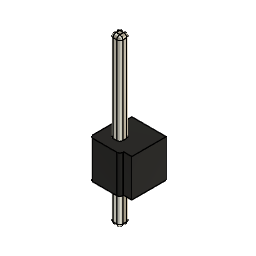
Parametric_Male (Autodesk Fusion 360 design; units mm, degrees)
Autodesk Fusion 360 part; units mm, degrees
sketch "Sketch1" plane through (0, 0, 0) normal (0, 0, 1) x (1, 0, 0)
  line L0 (1, -1) -> (-1, -1)
  line L1 (-1, -1) -> (-1, 1)
  line L2 (-1, 1) -> (1, 1)
  line L3 (1, 1) -> (1, -1)
  line L4 (1, -1) -> (-1, 1) construction
  line L5 (-1, -1) -> (1, 1) construction
  line L6 (0.325, -0.325) -> (-0.325, -0.325)
  line L7 (-0.325, -0.325) -> (-0.325, 0.325)
  line L8 (-0.325, 0.325) -> (0.325, 0.325)
  line L9 (0.325, 0.325) -> (0.325, -0.325)
  line L10 (0.325, -0.325) -> (-0.325, 0.325) construction
  line L11 (-0.325, -0.325) -> (0.325, 0.325) construction
  line L12 (1, 0.75) -> (1.54, 0.75)
  line L13 (1.54, 0.75) -> (1.54, -0.75)
  line L14 (1.54, -0.75) -> (1, -0.75)
  line L15 (1, -0.75) -> (1, 0.75)
  line L16 (-0.75, 1) -> (0.75, 1)
  line L17 (0.75, 1) -> (0.75, 1.54)
  line L18 (0.75, 1.54) -> (-0.75, 1.54)
  line L19 (-0.75, 1.54) -> (-0.75, 1)
  line L20 (0.75, 1.54) -> (1.54, 1.54)
  line L21 (1.54, 1.54) -> (1.54, 0.75)
  dimension "d1" = 2
  dimension "d2" = 2
  dimension "d5" = 0.65
  dimension "d6" = 0.65
  dimension "d13" = 0.54
  dimension "d14" = 0.25
  dimension "d15" = 0.25
  dimension "d16" = 0.54
  dimension "d17" = 0.25
  dimension "d18" = 0.25
  constraint horizontal L0
  constraint perpendicular L0 L1
  constraint parallel L0 L2
  constraint parallel L1 L3
  constraint coincident L4 origin
  constraint coincident L5 origin
  constraint horizontal L6
  constraint perpendicular L6 L7
  constraint parallel L6 L8
  constraint parallel L7 L9
  constraint coincident L10 origin
  constraint coincident L11 origin
  constraint horizontal L12
  constraint vertical L13
  constraint horizontal L14
  constraint vertical L15
  constraint coincident L3 L12.start
  constraint horizontal L16
  constraint vertical L17
  constraint horizontal L18
  constraint vertical L19
  constraint coincident L2 L16.start
  constraint perpendicular L13 L20
  constraint perpendicular L12 L21
  measures "d1" distance of L1.end L2.end
  measures "d2" distance of L0.end L1.end
  measures "d5" distance of L7.end L8.end
  measures "d6" distance of L6.end L7.end
  measures "d13" distance of L12.start L12.end
  measures "d14" distance of L2 L12
  measures "d15" distance of L0 L14
  measures "d16" distance of L16.start L18.end
  measures "d17" distance of L1 L19
  measures "d18" distance of L3 L17
extrude "Extrude1" add sketch "Sketch1" along normal blind 2.5 contours L0 L1 L2 L3 L15 L16 | L3 L12 L13 L14 L15 | L2 L3 L12 L17 L20 L21 | L2 L16 L17 L18 L19 | L6 L7 L8 L9
extrude "Extrude2" add sketch "Sketch1" along normal blind 8.5 contours L6 L7 L8 L9
extrude "Extrude3" add sketch "Sketch1" against normal blind 2.5 contours L6 L7 L8 L9
fillet "Fillet1" radius 0.2 11 edges at (-0.325, -0.325, 5.5) (0.325, -0.325, 5.5) (-0.325, 0.325, 5.5) (0.325, 0.325, 5.5) (-1, -1, 1.25) (-1, 1, 1.25) (1, -1, 1.25) (-0.325, -0.325, -1.25) (-0.325, 0.325, -1.25) (0.325, -0.325, -1.25) (0.325, 0.325, -1.25) 2 faces at (0.1083, -0.1083, 8.5) (0.1083, -0.1083, -2.5)
pattern_linear "R-Pattern8" count 1 spacing 2.54 along (0, 1, 0) of "Extrude1", "Extrude2", "Extrude3", "Fillet1"
equation "d15 = d14"
equation "d17 = d14"
equation "d18 = d15"
equation "width = 1"
equation "length = 1"
equation "d61 = length"
equation "d62 = width"
named bodies: "Parametric_Male"
